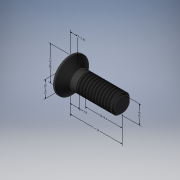
# Autodesk Inventor part: Senkschraube DIN ≈965 M5x14 51305.050.014(High)
Saved by Autodesk Inventor 2019 (Build 230136000, 136)
## iProperties
Created: 2022-09-09
Part Number: Senkschraube DIN ≈965 M5x14 51305.050.014(High)
Material: Generic
Catalog Web Link: www.cadenas.de
Description: DIN ≈965-Counter sunk screws with torx
Vendor: FABORY
Document SubType Name: Modeling
Designer: psAdmin
Manufacturer: FABORY
Mass: 2 g
Surface Area: 3.77256 cm^2
Volume: 0.306542 cm^3
Density: 1 g/cm^3
Appearance: PSOLRGB-175-175-175
Category: PARTsolutions
Company: FABORY
Title: Senkschraube DIN ≈965 M5x14
Author: Cadenas PARTsolutions
Comments: Counter sunk screws with torx
PSOL_IDENT_0: {$CADENAS_DATA/23d-libs/fabory/6_screws/din_965_v2.prj},222 {VTYP=3D},{NB=Senkschraube DIN ≈965 M5x1
PSOL_IDENT_1: 4 51305.050.014(High)},{LINA=Senkschraube DIN ≈965 M5x14},{NN=DIN ≈965},{DATE=02.05.2022 11:12:59},{
PSOL_IDENT_2: GEOMDATE=13.03.2019 09:47:59},{VERSION=},{LINEID=54320},{WBVAR=LOD},{WBNUMERIC=}  {NB=Senkschraube D
PSOL_IDENT_3: IN ≈965 M5x14 51305.050.014(High)},{LINA=Senkschraube DIN ≈965 M5x14},{KT=DUMMY},{CNSORDERNO=51305.0
PSOL_IDENT_4: 50.014},{NENNID=M5x14},{D=5.000},{L=14},{ERPPDMNUMBER=51305.050.014},{BRAND=Fabory},{STANDARD=DIN ≈9
PSOL_IDENT_5: 65},{THREAD=Metric thread},{THREADDIRECTION=},{STYLE=},{TYPE=Machine screw},{GRADE=A2},{BASICMATERIA
PSOL_IDENT_6: L=Stainless steel},{SURFACETREATMEN=},{HEADSHAPE=Countersunk head},{DRIVINGFEATURE=Hexalobular},{CNS
PSOL_IDENT_7: MASSEXACT=0.00219},{COLOR=},{COMPARABLESTAND=ISO≈14581;NF≈E25-119-1},{ADDITIONALINFO=Metric},{ROHS=Y
PSOL_IDENT_8: },{APPROVAL=},{EANCODE=8715494281416},{INTRASTCODE=},{ECLASS=},{UNSPSC=31161504},{ETIM=EC000887},{UR
PSOL_IDENT_9: L=https://www.fabory.com/en-GB/p/51305050014},{PACKAGING=MIN},{VARIANT=MIN},{FABNENN=},{FABGEO=},{FA
PSOL_IDENT_10: BARTICLENR=51305.050.014},{FABNETWEIGHT=2.190},{NENN=M5x14},{D3=4.019},{P=0.800},{DIN962THREAD=},{XL
PSOL_IDENT_11: H=0},{DIN962OPT2=},{OPTIONS2L='',' - ','din_962_std_mid.jpg','-S','S Splintloch','din_962_s_1.jpg'},
PSOL_IDENT_12: {DIN962OPT3=},{OPTIONSS='',' - ','din_962_std_gew.jpg','-SC','SC Schabenut','din_962_sc.jpg','-FL','
PSOL_IDENT_13: FL Kegelstumpf','din_962_fl.jpg','-CN','CN Spitze','din_962_cn.jpg','-CH','CH Kegelkuppe','din_962_c
PSOL_IDENT_14: h.jpg','-CP','CP Ringschneide','din_962_cp.jpg','-RL','RL ohne Kuppe','din_962_rl.jpg','-RN','RN Lin
PSOL_IDENT_15: senkuppe','din_962_rn.jpg','-SD','SD Kurzer Zapfen','din_962_sd.jpg','-LD','LD Lange Zapfen','din_96
PSOL_IDENT_16: 2_ld.jpg'},{B=9.900},{B2=25.000},{A1=1.600},{DK=9.20},{K=2.500},{R=0.500},{X=1.75},{NR=25},{A=4.50},
PSOL_IDENT_17: {T=1.91},{NRP=MIN},{M=MIN},{SCLN=4},{SCDN=3.72},{SCLK=2.4},{Z0H=1},{Z0D2=9},{Z1H=1},{Z1D2=10},{Z2H=1
PSOL_IDENT_18: .6},{Z2D2=15},{SD1=1.2},{SLE=2.6},{FLDP=3.5},{CPDZ=2.5},{TCDT=0},{SDDP=3.5},{SDZ1=1.25},{LDDP=3.5},{
PSOL_IDENT_19: LDZ2=2.5},{DIN962FTHREAD=0},{VERS=2},{CNSAVOID=0},{DIST=0.464},{LINK1=51305},{LINK2=050},{LINK3=014}
PSOL_IDENT_20: ,{INFOPATH=https://www.fabory.com/en-GB/p/51305050014},{LOD=High},{STANDARDSMALL=din_965_v2.png}
NB: Senkschraube DIN ≈965 M5x14 51305.050.014(High)
NN: DIN ≈965
NT: Counter sunk screws with torx
NBSYN: Senkschraube DIN ≈965 $NENN. $CNSORDERNO.($LOD.)
LINA: Senkschraube DIN ≈965 M5x14
CATALOG: Fabory
ROWDESC: M5x14
OFFICIAL_STANDARD_NUMBERS: ISO 14581
CNSORDERNO: 51305.050.014
NENNID: M5x14
D: 5
L: 14
BRAND: Fabory
STANDARD: DIN ≈965
THREAD: Metric thread
TYPE: Machine screw
GRADE: A2
BASICMATERIAL: Stainless steel
HEADSHAPE: Countersunk head
DRIVINGFEATURE: Hexalobular
CNSMASSEXACT: 0.002
COMPARABLESTAND: ISO≈14581;NF≈E25-119-1
ROHS: Y
EANCODE: 8715494281416
UNSPSC: 31161504
ETIM: EC000887
URL: https://www.fabory.com/en-GB/p/51305050014
D3: 4.019
P: 0.8
B: 9.9
B2: 25
A1: 1.6
DK: 9.2
K: 2.5
R: 0.5
X: 1.75
NR: 25
A: 4.5
T: 1.91
NRP: 0
M: 0
SUPPLIER: FABORY
ARTICLENO: Senkschraube DIN ≈965 M5x14 51305.050.014(High)
BOMINFO: Senkschraube DIN ≈965 M5x14
CREATOR: CADENAS GmbH
Autodesk Inventor part; units mm, degrees
sketch "Skizze_5" plane through (0, 0, 0) normal (0, 0, 1) x (1, 0, 0)
  line L0 (14, 0) -> (0, 0)
  line L1 (0, 0) -> (0, 4.6)
  line L2 (0, 4.6) -> (0.4, 4.6)
  line L3 (0.4, 4.6) -> (2.5, 2.5)
  line L4 (2.5, 2.5) -> (13.5095, 2.5)
  line L5 (13.5095, 2.5) -> (14, 2.0095)
  line L6 (14, 2.0095) -> (14, 0)
  line L7 (14, 0) -> (0, 0)
  constraints: 16 end point
revolve "Revolution1" add sketch "Skizze_5" angle 360 about axis through (14, 0, 0) along (1, 0, 0)
thread "Thread1" size "M5x0.8" class "6g" standard "ISO Metric profile" length 9.4095
sketch "Sketch_1" plane through (0, 0, 0) normal (0, 0, 1) x (1, 0, 0)
  line L0 (1.91, 0) -> (0, 0)
  line L1 (0, 0) -> (0, 2.25)
  line L2 (0, 2.25) -> (1.91, 2.25)
  line L3 (1.91, 2.25) -> (1.91, 0)
  line L4 (1.91, 0) -> (0, 0)
  constraints: 10 end point
revolve "Revolution2" cut sketch "Sketch_1" angle 360 about axis through (1.91, 0, 0) along (1, 0, 0)
sketch "Sketch_2" plane through (0, 0, 0) normal (0, 0, 1) x (1, 0, 0)
  line L0 (3.209, 0) -> (1.91, 0)
  line L1 (1.91, 0) -> (1.91, 2.25)
  line L2 (1.91, 2.25) -> (3.209, 0)
  line L3 (3.209, 0) -> (1.91, 0)
  constraints: 8 end point
revolve "Revolution3" cut sketch "Sketch_2" angle 360 about axis through (3.209, 0, 0) along (1, 0, 0)
sketch "Sketch_3" plane through (0, 0, 0) normal (1, 0, 0) x (0, 1, 0)
  circle A0 centre (0, 0) radius 2.7
  arc A1 (-0.5727, 1.8677) -> (-1.3311, 1.4298) centre (-0.9, 1.5588) ccw
  arc A2 (-1.9038, 0.4379) -> (-1.3311, 1.4298) centre (-2.0856, 1.2041) ccw
  arc A3 (-1.9038, 0.4379) -> (-1.9038, -0.4379) centre (-1.8, 0) ccw
  arc A4 (-1.3311, -1.4298) -> (-1.9038, -0.4379) centre (-2.0856, -1.2041) ccw
  arc A5 (-1.3311, -1.4298) -> (-0.5727, -1.8677) centre (-0.9, -1.5588) ccw
  arc A6 (0.5727, -1.8677) -> (-0.5727, -1.8677) centre (0, -2.4082) ccw
  arc A7 (0.5727, -1.8677) -> (1.3311, -1.4298) centre (0.9, -1.5588) ccw
  arc A8 (1.9038, -0.4379) -> (1.3311, -1.4298) centre (2.0856, -1.2041) ccw
  arc A9 (1.9038, -0.4379) -> (1.9038, 0.4379) centre (1.8, 0) ccw
  arc A10 (1.3311, 1.4298) -> (1.9038, 0.4379) centre (2.0856, 1.2041) ccw
  arc A11 (1.3311, 1.4298) -> (0.5727, 1.8677) centre (0.9, 1.5588) ccw
  arc A12 (-0.5727, 1.8677) -> (0.5727, 1.8677) centre (0, 2.4082) ccw
  constraints: 24 point on circle, 13 centre point
extrude "Extrusion1" add sketch "Sketch_3" along normal blind 1.91
sketch "Sketch_4" plane through (0, 0, 0) normal (0, 0, 1) x (1, 0, 0)
  line L0 (1.299, 0) -> (-1.91, 0)
  line L1 (-1.91, 0) -> (-1.91, 2.25)
  line L2 (-1.91, 2.25) -> (0, 2.25)
  line L3 (0, 2.25) -> (1.299, 0)
  line L4 (1.299, 0) -> (-1.91, 0)
  constraints: 10 end point
revolve "Revolution4" cut sketch "Sketch_4" angle 360 about axis through (1.299, 0, 0) along (1, 0, 0)
ref_plane "IP1_XY" through (0, 0, 0) normal (1, 0, 0) x (0, 0, -1)
ref_plane "IP1_YZ" through (0, 0, 0) normal (0, 0, -1) x (0, 1, 0)
ref_plane "IP1_ZX" through (0, 0, 0) normal (0, 1, 0) x (1, 0, 0)
ref_plane "IP2_XY" through (2.5, 0, 0) normal (1, 0, 0) x (0, 0, -1)
ref_plane "IP2_YZ" through (2.5, 0, 0) normal (0, 0, -1) x (0, 1, 0)
ref_plane "IP2_ZX" through (2.5, 0, 0) normal (0, 1, 0) x (1, 0, 0)
ref_plane "IP3_XY" through (14, 0, 0) normal (1, 0, 0) x (0, 0, -1)
ref_plane "IP3_YZ" through (14, 0, 0) normal (0, 0, -1) x (0, 1, 0)
ref_plane "IP3_ZX" through (14, 0, 0) normal (0, 1, 0) x (1, 0, 0)
body "Solid1"
